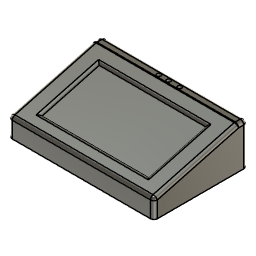
Sketch 3.1 v5 (Autodesk Fusion 360 design; units mm, degrees)
Autodesk Fusion 360 part; units mm, degrees
sketch "Sketch1" plane through (0, 0, 0) normal (0, 0, 1) x (1, 0, 0)
  line L0 (-100.0661, 42.8855) -> (109.9339, 42.8855)
  line L1 (109.9339, 42.8855) -> (109.9339, -80.1145)
  line L2 (109.9339, -80.1145) -> (-100.0661, -80.1145)
  line L3 (-100.0661, -80.1145) -> (-100.0661, 42.8855)
  dimension "d1" = 210
  dimension "d2" = 123
  constraint horizontal L0
  constraint vertical L1
  constraint horizontal L2
  constraint vertical L3
  measures "d1" distance of L0.start L0.end
  measures "d2" distance of L0.start L2.end
extrude "Extrude1" add sketch "Sketch1" along normal blind 60 makes body 1
chamfer "Chamfer1" distance 122 angle 15 1 edges at (4.9339, -80.1145, 60) measured on face at (-30.0661, -39.1145, 60) on bodies 1
extrude "Extrude2" add 1 faces at (-30.0661, 42.8855, 20) along direction (0, 1, 0) blind 2 on bodies 1 bodies 1
shell "Shell1" thickness 3 removed faces 0 bodies 1
sketch "Sketch2" plane through (0, 0, 0) normal (0, 0, -1) x (1, 0, 0)
  line L0 (109.9339, 80.1145) -> (-100.0661, 80.1145)
  line L1 (-100.0661, 80.1145) -> (-100.0661, -44.8855)
  line L2 (-100.0661, -44.8855) -> (109.9339, -44.8855)
  line L3 (109.9339, -44.8855) -> (109.9339, 80.1145)
  line L4 (106.9339, -40.8855) -> (-97.0661, -40.8855)
  line L5 (-97.0661, -40.8855) -> (-97.0661, 76.1145)
  line L6 (-97.0661, 76.1145) -> (106.9339, 76.1145)
  line L7 (106.9339, 76.1145) -> (106.9339, -40.8855)
  dimension "d10" = 204
  dimension "d11" = 117
  dimension "d12" = 3
  dimension "d13" = 210
  dimension "d14" = 4
  constraint horizontal L4
  constraint vertical L5
  constraint horizontal L6
  constraint vertical L7
  measures "d10" distance of L4.start L4.end
  measures "d11" distance of L4.start L6.end
  measures "d12" distance of L1 L5
  measures "d13" distance of L1.end L2.end
  measures "d14" distance of L0 L6
extrude "Extrude3" cut sketch "Sketch2" against normal blind 3 contours L4 L5 L6 L7 bodies 1
extrude "Extrude4" cut 1 faces at (38.9339, 40.8855, 1) along direction (0, 1, 0) blind 1 on bodies 1 bodies 1
extrude "Extrude5" cut 1 faces at (-29.0661, -76.1145, 1) along direction (0, -1, 0) blind 1 on bodies 1 bodies 1
sketch "Sketch3" plane through (0, -12.1942, 45.5094) normal (0, -0.258819, 0.965926) x (1, 0, 0)
  line L0 (109.9339, -70.3163) -> (109.9339, 55.9874)
  line L1 (109.9339, 55.9874) -> (-100.0661, 55.9874)
  line L2 (-100.0661, 55.9874) -> (-100.0661, -70.3163)
  line L3 (-100.0661, -70.3163) -> (109.9339, -70.3163)
  line L4 (-72.5661, 35.8357) -> (82.4339, 35.8357)
  line L5 (82.4339, 35.8357) -> (82.4339, -50.1643)
  line L6 (82.4339, -50.1643) -> (-72.5661, -50.1643)
  line L7 (-72.5661, -50.1643) -> (-72.5661, 35.8357)
  dimension "d21" = 155
  dimension "d22" = 86
  dimension "d23" = 20.152
  dimension "d73" = 126.3037
  dimension "d74" = 27.5
  dimension "d75" = 27.5
  dimension "d76" = 20.1517
  constraint horizontal L4
  constraint vertical L5
  constraint horizontal L6
  constraint vertical L7
  measures "d21" distance of L4.start L4.end
  measures "d22" distance of L4.start L6.end
  measures "d23" distance of L3 L6
  measures "d73" distance of L1.end L2.end
  measures "d74" distance of L2 L7
  measures "d75" distance of L0 L5
  measures "d76" distance of L1 L4
extrude "Extrude6" cut sketch "Sketch3" against normal blind 3 contours L4 L5 L6 L7 bodies 1
fillet "Fillet1" radius 4 1 edges at (-72.5661, -19.1144, 43.6551) on bodies 1
fillet "Fillet2" radius 4 1 edges at (2.9974, -60.6492, 32.5259) on bodies 1
fillet "Fillet3" radius 4 1 edges at (2.9974, 22.4204, 54.7844) on bodies 1
fillet "Fillet4" radius 4 1 edges at (82.4339, -19.1144, 43.6551) on bodies 1
extrude "Extrude7" add 1 faces at (-97.0661, 2.2188, 27.3008) along direction (1, 0, 0) blind 3 on bodies 1 bodies 1
extrude "Extrude8" add 1 faces at (106.9339, 2.2188, 27.3008) along direction (-1, 0, 0) blind 3 on bodies 1 bodies 1
extrude "Extrude9" add 1 faces at (-28.0661, -77.1145, 16.6721) along direction (0, 1, 0) blind 3 on bodies 1 bodies 1
extrude "Extrude10" add 1 faces at (-28.0661, 41.8855, 37.9294) along direction (0, -1, 0) blind 3 on bodies 1 bodies 1
sketch "Sketch4" plane through (0, 0, 0) normal (0, 0, -1) x (1, 0, 0)
  line L0 (109.9339, 80.1145) -> (-100.0661, 80.1145)
  line L1 (-100.0661, 80.1145) -> (-100.0661, -44.8855)
  line L2 (-100.0661, -44.8855) -> (109.9339, -44.8855)
  line L3 (109.9339, -44.8855) -> (109.9339, 80.1145)
  line L4 (-94.0661, 74.1145) -> (103.9339, 74.1145)
  line L5 (103.9339, 74.1145) -> (103.9339, -38.8855)
  line L6 (103.9339, -38.8855) -> (-94.0661, -38.8855)
  line L7 (-94.0661, -38.8855) -> (-94.0661, 74.1145)
  line L8 (106.9339, -41.8855) -> (-97.0661, -41.8855)
  line L9 (-97.0661, -41.8855) -> (-97.0661, 77.1145)
  line L10 (-97.0661, 77.1145) -> (106.9339, 77.1145)
  line L11 (106.9339, 77.1145) -> (106.9339, -41.8855)
  dimension "d42" = 204
  dimension "d43" = 119
  dimension "d44" = 3
  dimension "d45" = 3
  constraint horizontal L8
  constraint vertical L9
  constraint horizontal L10
  constraint vertical L11
  measures "d42" distance of L8.start L8.end
  measures "d43" distance of L8.start L10.end
  measures "d44" distance of L3 L11
  measures "d45" distance of L2 L8
extrude "Extrude11" cut sketch "Sketch4" against normal blind 3 contours L8 L9 L10 L11 bodies 1
hole "Hole1" at (-100.0661, 27.4404, 22.7342) direction (1, 0, 0) diameter 10 depth 10 tip angle 180 bodies 1
move_face "MoveFace1" to x (1, 0, 0) y (0, 1, 0) z (0, 0, 1) at (0, -9.2, -2) 5 faces at (-96.0661, 27.9383, 27.7094) (-100.0661, -4.7298, 37.9032) (103.9339, 1.2188, 28.0328) (-94.0661, -3.8993, 35.6501) (109.9339, 2.2188, 29.1034) on bodies 1
extrude "Extrude12" add 1 faces at (-30.0661, 44.8855, 20) along direction (0, 1, 0) blind 10 on bodies 1 bodies 1
extrude "Extrude13" cut 1 faces at (38.9339, 41.8855, 1) along direction (0, 1, 0) blind 10 on bodies 1 bodies 1
extrude "Extrude14" cut 1 faces at (-28.0661, 38.8855, 38.3935) along direction (0, 1, 0) blind 10 on bodies 1 bodies 1
fillet "Fillet5" radius 5 1 edges at (109.9339, 54.8855, 30) on bodies 1
fillet "Fillet6" radius 5 3 edges at (2.4339, 54.8855, 60) (108.4694, 53.421, 60) (109.9339, 45.8855, 60) on bodies 1
fillet "Fillet7" radius 5 3 edges at (109.9339, -28.4447, 41.1551) (108.4694, 36.42, 58.5355) (2.4339, 41.8855, 60) on bodies 1
fillet "Fillet8" radius 5 3 edges at (2.4339, -80.1145, 27.3102) (108.4694, -80.1145, 25.7941) (109.9339, -80.1145, 11.0669) on bodies 1
fillet "Fillet9" radius 5 7 edges at (-100.0661, 54.8855, 27.5) (-100.0661, 53.421, 58.5355) (-100.0661, 46.2146, 60) (-100.0661, 41.8911, 59.9572) (-100.0661, -17.5795, 44.0664) (-100.0661, -79.0813, 26.5174) (-100.0661, -80.1145, 11.7368) on bodies 1
sketch "Sketch5" plane through (0, 0, 60) normal (0, 0, 1) x (-1, 0, 0)
  line L0 (95.0661, -49.8855) -> (95.0661, -42.5437)
  line L1 (95.0661, -42.5437) -> (-104.9339, -42.5437)
  line L2 (-104.9339, -42.5437) -> (-104.9339, -49.8855)
  line L3 (-104.9339, -49.8855) -> (95.0661, -49.8855)
  circle A0 centre (-21.0687, -46.2251) radius 3
  circle A1 centre (-21.0687, -46.2251) radius 3
  circle A2 centre (9.3174, -46.3343) radius 3
  circle A3 centre (-4.9339, -46.3343) radius 3
  dimension "d67" = 6
  dimension "d68" = 6
  dimension "d69" = 6
  dimension "d70" = 6
  constraint concentric A0 A1
  measures "d67" diameter of A0
  measures "d68" diameter of A1
  measures "d69" diameter of A2
  measures "d70" diameter of A3
extrude "Extrude15" cut sketch "Sketch5" against normal blind 5 contours A0 A1 | A2 | A3 bodies 1
sketch "Sketch6" plane through (0, 0, 0) normal (0, 0, 1) x (1, 0, 0)
  line L0 (-91, -110) -> (85, -110)
  line L1 (94, -119) -> (94, -211)
  line L2 (85, -220) -> (-91, -220)
  line L3 (-100, -211) -> (-100, -119)
  arc A0 (-91, -110) -> (-100, -119) centre (-91, -119) ccw
  arc A1 (-100, -211) -> (-91, -220) centre (-91, -211) ccw
  arc A2 (85, -220) -> (94, -211) centre (85, -211) ccw
  arc A3 (94, -119) -> (85, -110) centre (85, -119) ccw
  point P0 (-100, -110)
  point P1 (94, -110)
  point P2 (-100, -220)
  dimension "d77" = 194
  dimension "d78" = 110
  dimension "d79" = 9
  dimension "d80" = 9
  dimension "d81" = 9
  dimension "d82" = 9
  constraint horizontal L0
  constraint vertical L1
  constraint horizontal L2
  constraint vertical L3
  constraint coincident P0 L0
  constraint coincident P0 L3
  constraint tangent L0 A0
  constraint tangent L3 A0
  constraint coincident P2 L2
  constraint coincident P2 L3
  constraint tangent L2 A1
  constraint tangent L3 A1
  constraint tangent L1 A2
  constraint tangent L2 A2
  constraint coincident P1 L0
  constraint coincident P1 L1
  constraint tangent L0 A3
  constraint tangent L1 A3
  measures "d77" distance of P0 P1
  measures "d78" distance of P0 P2
  measures "d79" radius of A0
  measures "d80" radius of A1
  measures "d81" radius of A2
  measures "d82" radius of A3
extrude "Extrude16" add sketch "Sketch6" along normal blind 20 separate body makes body 2
move_body "Move1" bodies 2 to x (1, 0, 0) y (0, 1, 0) z (0, 0, 1) at (0, 70, 0)
move_body "Move2" bodies 2 to x (1, 0, 0) y (0, 0.965926, 0.258819) z (0, -0.258819, 0.965926) at (0, 94.8889, 38.8229)
move_body "Move3" bodies 2 to x (1, 0, 0) y (0, 1, 0) z (0, 0, 1) at (10, 0, 0)
move_body "Move4" bodies 2 to x (1, 0, 0) y (0, 1, 0) z (0, 0, 1) at (0, -10, 5)
move_body "Move5" bodies 2 to x (1, 0, 0) y (0, 1, 0) z (0, 0, 1) at (-3.0044, -6.6388, 0)
move_body "Move6" bodies 2 to x (1, 0, 0) y (0, 1, 0) z (0, 0, 1) at (0, 0, -2.7)
move_face "MoveFace2" by (1, 0, 0) 1 faces at (-25.3377, -36.3979, 31.1085) on bodies 2
move_body "Move7" bodies 2 to x (1, 0, 0) y (0, 1, 0) z (0, 0, 1) at (1, 0, 0)
move_body "Move8" bodies 2 to x (1, 0, 0) y (0, 1, 0) z (0, 0, 1) at (0, 0, 5)
sketch "Sketch8" plane through (0, 0, 3) normal (0, 0, -1) x (1, 0, 0)
  line L0 (106.9339, 77.1145) -> (-97.0661, 77.1145)
  line L1 (-97.0661, 77.1145) -> (-97.0661, -51.8855)
  line L2 (-97.0661, -51.8855) -> (106.9339, -51.8855)
  line L3 (106.9339, -51.8855) -> (106.9339, 77.1145)
  line L4 (103.9339, 74.1145) -> (103.9339, -48.8855)
  line L5 (103.9339, -48.8855) -> (-94.0661, -48.8855)
  line L6 (-94.0661, -48.8855) -> (-94.0661, 74.1145)
  line L7 (-94.0661, 74.1145) -> (103.9339, 74.1145)
  line L8 (-97.0661, 77.1145) -> (106.7339, 77.1145)
  line L9 (106.7339, 77.1145) -> (106.7339, -51.6855)
  line L10 (106.7339, -51.6855) -> (-97.0661, -51.6855)
  line L11 (-97.0661, -51.6855) -> (-97.0661, 77.1145)
  dimension "d85" = 203.8
  dimension "d86" = 128.8
  constraint horizontal L8
  constraint vertical L9
  constraint horizontal L10
  constraint vertical L11
  constraint coincident L0.end L1.start
  measures "d85" distance of L0.end L8.end
  measures "d86" distance of L0.end L10.end
extrude "Extrude17" add sketch "Sketch8" along normal blind 2.95 separate body contours L0 L1 L8 L9 L10 L11 | L4 L5 L6 L7 makes body 3
hole "Hole2" at (-95.2768, 49.8187, 0.05) direction (0, 0, 1) diameter 2 depth 16 tip angle 180 bodies 1 3
hole "Hole3" at (-95.2409, -75.4084, 0.05) direction (0, 0, 1) diameter 2 depth 16 tip angle 180 bodies 1 3
hole "Hole4" at (104.9038, 49.9588, 0.05) direction (0, 0, 1) diameter 2 depth 16 tip angle 180 bodies 1 3
hole "Hole5" at (105.1009, -75.3485, 0.05) direction (0, 0, 1) diameter 2 depth 16 tip angle 180 bodies 1 3
sketch "Sketch9" plane through (0, 0, 3) normal (0, 0, -1) x (1, 0, 0)
  line L0 (-94.0295, -48.8484) -> (103.8838, -48.8484)
  line L1 (103.8838, -48.8484) -> (103.8838, 74.0653)
  line L2 (103.8838, 74.0653) -> (-94.0295, 74.0653)
  line L3 (-94.0295, 74.0653) -> (-94.0295, -48.8484)
  constraint horizontal L0
  constraint vertical L1
  constraint horizontal L2
  constraint vertical L3
extrude "Extrude18" add sketch "Sketch9" against normal blind 52.9 separate body makes body 4
chamfer "Chamfer2" distance 111 distance2 29.8 1 edges at (4.9271, -74.0653, 55.9) measured on face at (37.9127, 7.8772, 55.9) on bodies 4
sketch "Sketch10" plane through (103.8838, 0, 0) normal (1, 0, 0) x (0, 1, 0)
  line L0 (36.9347, 55.9) -> (-74.0653, 26.1)
  line L1 (-74.0653, 26.1) -> (-74.0653, 3)
  line L2 (-74.0653, 3) -> (48.8484, 3)
  line L3 (48.8484, 3) -> (48.8484, 55.9)
  line L4 (48.8484, 55.9) -> (36.9347, 55.9)
  line L5 (39.6042, 35.7447) -> (39.6042, 3)
  line L6 (-66.6959, 3) -> (-66.6959, 7.2332)
  line L7 (-66.6959, 7.2332) -> (39.6042, 35.7447)
  constraint coincident L2 L5.end
  constraint perpendicular L2 L5
  constraint coincident L2 L6.start
  constraint perpendicular L2 L6
extrude "Extrude19" cut sketch "Sketch10" against normal blind 220 contours L2 L5 L6 L7 bodies 4
sketch "Sketch11" plane through (103.8838, 0, 0) normal (1, 0, 0) x (0, 1, 0)
  line L0 (-66.6959, 3) -> (-66.6959, 7.2332)
  line L1 (-66.6959, 7.2332) -> (39.6042, 35.7447)
  line L2 (39.6042, 35.7447) -> (39.6042, 3)
  line L3 (39.6042, 3) -> (48.8484, 3)
  line L4 (48.8484, 3) -> (48.8484, 55.9)
  line L5 (48.8484, 55.9) -> (36.9347, 55.9)
  line L6 (36.9347, 55.9) -> (-74.0653, 26.1)
  line L7 (-74.0653, 26.1) -> (-74.0653, 3)
  line L8 (-74.0653, 3) -> (-66.6959, 3)
  line L9 (39.6042, 35.7447) -> (34.3774, 55.2135)
  line L10 (-71.8457, 26.6959) -> (-66.6302, 7.2508)
  constraint coincident L1.end L2.start
  constraint coincident L6 L9.end
  constraint perpendicular L6 L9
  constraint coincident L6 L10.start
  constraint coincident L1 L10.end
  constraint perpendicular L1 L10
sketch "Sketch12" plane through (0, 0, 0) normal (0, 0, 1) x (1, 0, 0)
sketch "Sketch13" plane through (0, 0, 0) normal (1, 0, 0) x (0, 1, 0)
  line L0 (39.654, 35.7144) -> (39.654, 31.4601)
  line L1 (39.654, 31.4601) -> (-66.7, 3)
  line L2 (-66.7, 3) -> (-66.7, 7.2353)
  line L3 (-66.7, 7.2353) -> (39.654, 35.7144)
  constraint vertical L0
  constraint parallel L0 L2
move_body "Move9" bodies 2 to x (1, 0, 0) y (0, 1, 0) z (0, 0, 1) at (0, 0, 50)
extrude "Extrude20" cut sketch "Sketch11" against normal blind 220 contours L1 L6 L9 L10 bodies 4 makes body 5 at (37.9127, 48.8484, 20.6333)
move_body "Move11" bodies 2 to x (1, 0, 0) y (0, 1, 0) z (0, 0, 1) at (0, 0, -50)
move_body "Move12" bodies 3 to x (1, 0, 0) y (0, 1, 0) z (0, 0, 1) at (0, 0, -10)
extrude "Extrude21" add sketch "Sketch13" along normal blind 104 and the other way blind 94 bodies 4 3 5
sketch "Sketch14" plane through (0, -6.2705, 23.4169) normal (0, -0.258664, 0.965967) x (1, 0, 0)
  line L0 (103.8838, -62.487) -> (103.8838, -62.5585)
  line L1 (103.8838, -62.5585) -> (104, -62.5585)
  line L2 (104, -62.5585) -> (104, 47.5425)
  line L3 (104, 47.5425) -> (103.8838, 47.5425)
  line L4 (103.8838, 47.5425) -> (103.8838, 47.4909)
  line L5 (103.8838, 47.4909) -> (-94, 47.4909)
  line L6 (-94, 47.4909) -> (-94, -62.487)
  line L7 (-94, -62.487) -> (103.8838, -62.487)
  line L8 (-50, 30) -> (60.2105, 30)
  line L9 (60.2105, 30) -> (60.2105, -45.8455)
  line L10 (60.2105, -45.8455) -> (-50, -45.8455)
  line L11 (-50, -45.8455) -> (-50, 30)
  dimension "d113" = 110.2105
  dimension "d114" = 75.8455
  constraint horizontal L8
  constraint vertical L9
  constraint horizontal L10
  constraint vertical L11
  measures "d113" distance of L8.start L8.end
  measures "d114" distance of L8.start L10.end
extrude "Extrude22" cut sketch "Sketch14" against normal blind 10 contours L8 L9 L10 L11 bodies 4
move_body "Move13" bodies 3 to x (1, 0, 0) y (0, 1, 0) z (0, 0, 1) at (0, 0, 10)
move_body "Move10" [rolled back]
named bodies: "Upper Case", "Screen+Pi", "Under Case", "Screen Holder", "Screen Holder (1)"
